Autodesk Fusion 360 part; units mm, degrees
(part 2 of 3)
sketch "Sketch3" plane through (0, 0, 0) normal (0, -1, 0) x (1, 0, 0)
  spline S0 degree 3 poles (-0.0363, -10.6479) (-0.1747, -12.1181) (-0.1574, -12.2391) (0.1193, -12.2391) knots -1 -1 -1 -1 0 0 0 0
  spline S1 degree 3 poles (0.0329, -8.3995) (0.0674, -8.7454) (0.0329, -9.7659) (-0.0363, -10.6479) knots -1 -1 -1 -1 0 0 0 0
  spline S2 degree 3 poles (0.6036, -7.6558) (-0.0363, -7.7596) (-0.0536, -7.7769) (0.0329, -8.3995) knots -1 -1 -1 -1 0 0 0 0
  spline S3 degree 3 poles (1.9872, -8.5379) (1.9872, -7.8288) (1.4857, -7.5002) (0.6036, -7.6558) knots -1 -1 -1 -1 0 0 0 0
  spline S4 degree 3 poles (2.091, -10.6479) (2.0391, -9.7832) (1.9872, -8.8319) (1.9872, -8.5379) knots -1 -1 -1 -1 0 0 0 0
  spline S5 degree 3 poles (1.8316, -12.2391) (2.1948, -12.2391) (2.2121, -12.1872) (2.091, -10.6479) knots -1 -1 -1 -1 0 0 0 0
  spline S6 degree 3 poles (1.4684, -11.5646) (1.4684, -12.1353) (1.5203, -12.2391) (1.8316, -12.2391) knots -1 -1 -1 -1 0 0 0 0
  spline S7 degree 3 poles (0.6901, -10.6825) (1.0879, -10.3539) (1.4684, -10.769) (1.4684, -11.5646) knots -1 -1 -1 -1 0 0 0 0
  spline S8 degree 3 poles (0.4306, -11.5646) (0.4306, -11.1841) (0.5344, -10.8036) (0.6901, -10.6825) knots -1 -1 -1 -1 0 0 0 0
  spline S9 degree 3 poles (0.1193, -12.2391) (0.3615, -12.2391) (0.4306, -12.1008) (0.4306, -11.5646) knots -1 -1 -1 -1 0 0 0 0
  spline S10 degree 3 poles (4.9966, -12.0835) (5.1869, -12.2737) (10.1161, -11.7548) (10.1161, -11.5473) knots -1 -1 -1 -1 0 0 0 0
  spline S11 degree 3 poles (4.9275, -11.4435) (4.9275, -11.7548) (4.962, -12.0489) (4.9966, -12.0835) knots -1 -1 -1 -1 0 0 0 0
  spline S12 degree 3 poles (5.4117, -10.942) (4.962, -10.8728) (4.9275, -10.9074) (4.9275, -11.4435) knots -1 -1 -1 -1 0 0 0 0
  spline S13 degree 3 poles (7.3488, -11.1149) (6.5359, -11.063) (5.6712, -10.9766) (5.4117, -10.942) knots -1 -1 -1 -1 0 0 0 0
  spline S14 degree 3 poles (10.1161, -11.5473) (10.1161, -11.3916) (9.2167, -11.236) (7.3488, -11.1149) knots -1 -1 -1 -1 0 0 0 0
  spline S15 degree 3 poles (-0.3304, -6.5316) (0.1885, -6.6873) (1.1916, -6.6008) (1.624, -6.3587) knots -1 -1 -1 -1 0 0 0 0
  spline S16 degree 3 poles (-1.9215, -5.0269) (-1.6275, -5.7187) (-0.9876, -6.3241) (-0.3304, -6.5316) knots -1 -1 -1 -1 0 0 0 0
  spline S17 degree 3 poles (-1.5929, -3.8681) (-2.2329, -4.1449) (-2.2674, -4.2313) (-1.9215, -5.0269) knots -1 -1 -1 -1 0 0 0 0
  spline S18 degree 3 poles (-0.4514, -2.4499) (-0.192, -2.7612) (-0.8146, -3.5568) (-1.5929, -3.8681) knots -1 -1 -1 -1 0 0 0 0
  spline S19 degree 3 poles (-1.5064, -2.6402) (-0.9184, -2.1386) (-0.7281, -2.104) (-0.4514, -2.4499) knots -1 -1 -1 -1 0 0 0 0
  spline S20 degree 3 poles (-3.7376, -2.571) (-3.0803, -3.2282) (-2.2328, -3.2455) (-1.5064, -2.6402) knots -1 -1 -1 -1 0 0 0 0
  spline S21 degree 3 poles (-4.2391, -1.81) (-4.2391, -1.9483) (-4.0143, -2.2943) (-3.7376, -2.571) knots -1 -1 -1 -1 0 0 0 0
  spline S22 degree 3 poles (-5.0693, -1.5851) (-4.7753, -1.2911) (-4.2391, -1.4295) (-4.2391, -1.81) knots -1 -1 -1 -1 0 0 0 0
  spline S23 degree 3 poles (-3.8932, -3.7471) (-4.7753, -3.2455) (-5.4671, -1.9829) (-5.0693, -1.5851) knots -1 -1 -1 -1 0 0 0 0
  spline S24 degree 3 poles (-4.8445, -5.4939) (-3.2187, -5.4939) (-2.6479, -4.4389) (-3.8932, -3.7471) knots -1 -1 -1 -1 0 0 0 0
  spline S25 degree 3 poles (-6.574, -4.387) (-7.1966, -4.6291) (-5.8476, -5.4939) (-4.8445, -5.4939) knots -1 -1 -1 -1 0 0 0 0
  spline S26 degree 3 poles (-6.3492, -3.9027) (-6.3146, -4.1276) (-6.401, -4.3351) (-6.574, -4.387) knots -1 -1 -1 -1 0 0 0 0
  spline S27 degree 3 poles (-7.0929, -3.5568) (-6.4875, -3.5049) (-6.401, -3.5568) (-6.3492, -3.9027) knots -1 -1 -1 -1 0 0 0 0
  spline S28 degree 3 poles (-10.2233, -1.7581) (-9.7045, -3.1071) (-8.7186, -3.6606) (-7.0929, -3.5568) knots -1 -1 -1 -1 0 0 0 0
  spline S29 degree 3 poles (-10.3098, -0.3053) (-10.4828, -0.876) (-10.4655, -1.1009) (-10.2233, -1.7581) knots -1 -1 -1 -1 0 0 0 0
  spline S30 degree 3 poles (-8.2171, 1.701) (-9.0645, 1.5626) (-10.0158, 0.6633) (-10.3098, -0.3053) knots -1 -1 -1 -1 0 0 0 0
  spline S31 degree 3 poles (-7.3523, 2.5312) (-7.041, 2.168) (-7.3869, 1.8394) (-8.2171, 1.701) knots -1 -1 -1 -1 0 0 0 0
  spline S32 degree 3 poles (-7.923, 2.8425) (-7.7155, 2.8079) (-7.4561, 2.6695) (-7.3523, 2.5312) knots -1 -1 -1 -1 0 0 0 0
  spline S33 degree 3 poles (-7.8366, 3.3613) (-8.3035, 2.8944) (-8.3035, 2.8944) (-7.923, 2.8425) knots -1 -1 -1 -1 0 0 0 0
  spline S34 degree 3 poles (-6.6778, 3.8456) (-7.1966, 3.8456) (-7.4734, 3.7246) (-7.8366, 3.3613) knots -1 -1 -1 -1 0 0 0 0
  line L0 (-6.6778, 3.8456) -> (-5.9687, 3.8456)
  line L1 (-5.9687, 3.8456) -> (-6.3319, 3.1711)
  spline S35 degree 3 poles (-6.1416, 1.5107) (-6.7297, 1.5107) (-6.7988, 2.2544) (-6.3319, 3.1711) knots -1 -1 -1 -1 0 0 0 0
  spline S36 degree 3 poles (-5.6055, 2.1161) (-5.7092, 1.6145) (-5.7957, 1.5107) (-6.1416, 1.5107) knots -1 -1 -1 -1 0 0 0 0
  spline S37 degree 3 poles (-5.0001, 3.1192) (-5.2595, 2.8944) (-5.5363, 2.4447) (-5.6055, 2.1161) knots -1 -1 -1 -1 0 0 0 0
  spline S38 degree 3 poles (-3.5646, 3.4651) (-4.3775, 3.517) (-4.6196, 3.4651) (-5.0001, 3.1192) knots -1 -1 -1 -1 0 0 0 0
  spline S39 degree 3 poles (-2.5442, 3.7764) (-2.5961, 3.4478) (-2.6825, 3.4132) (-3.5646, 3.4651) knots -1 -1 -1 -1 0 0 0 0
  spline S40 degree 3 poles (-4.3083, 4.5028) (-3.3052, 4.6066) (-2.475, 4.278) (-2.5442, 3.7764) knots -1 -1 -1 -1 0 0 0 0
  spline S41 degree 3 poles (-4.4121, 5.6962) (-5.813, 4.9525) (-5.7611, 4.3299) (-4.3083, 4.5028) knots -1 -1 -1 -1 0 0 0 0
  spline S42 degree 3 poles (-1.5929, 5.8519) (-2.4404, 6.2151) (-3.5646, 6.1459) (-4.4121, 5.6962) knots -1 -1 -1 -1 0 0 0 0
  spline S43 degree 3 poles (0.0847, 4.1223) (0.0847, 4.5028) (-0.9876, 5.6098) (-1.5929, 5.8519) knots -1 -1 -1 -1 0 0 0 0
  spline S44 degree 3 poles (0.8457, 3.6035) (0.5171, 3.4824) (0.0847, 3.7764) (0.0847, 4.1223) knots -1 -1 -1 -1 0 0 0 0
  spline S45 degree 3 poles (0.8457, 4.9179) (1.1916, 4.2261) (1.1916, 3.7418) (0.8457, 3.6035) knots -1 -1 -1 -1 0 0 0 0
  spline S46 degree 3 poles (0.863, 5.6789) (0.5863, 5.4714) (0.5863, 5.4195) (0.8457, 4.9179) knots -1 -1 -1 -1 0 0 0 0
  spline S47 degree 3 poles (3.4055, 6.0075) (2.7136, 6.1459) (1.2608, 5.973) (0.863, 5.6789) knots -1 -1 -1 -1 0 0 0 0
  spline S48 degree 3 poles (4.6334, 5.5406) (4.2702, 5.7308) (3.7168, 5.9384) (3.4055, 6.0075) knots -1 -1 -1 -1 0 0 0 0
  spline S49 degree 3 poles (4.9966, 4.866) (5.2907, 5.1947) (5.2907, 5.212) (4.6334, 5.5406) knots -1 -1 -1 -1 0 0 0 0
  spline S50 degree 3 poles (4.2875, 4.5374) (4.5124, 4.5374) (4.841, 4.6931) (4.9966, 4.866) knots -1 -1 -1 -1 0 0 0 0
  spline S51 degree 3 poles (2.5407, 3.811) (2.8347, 4.1396) (3.7687, 4.5374) (4.2875, 4.5374) knots -1 -1 -1 -1 0 0 0 0
  spline S52 degree 3 poles (2.8347, 2.9808) (2.4369, 2.9808) (2.2813, 3.4824) (2.5407, 3.811) knots -1 -1 -1 -1 0 0 0 0
  spline S53 degree 3 poles (3.44, 3.2403) (3.2671, 3.1019) (2.9904, 2.9808) (2.8347, 2.9808) knots -1 -1 -1 -1 0 0 0 0
  spline S54 degree 3 poles (6.2073, 2.2026) (5.9479, 3.2576) (4.2875, 3.8802) (3.44, 3.2403) knots -1 -1 -1 -1 0 0 0 0
  spline S55 degree 3 poles (6.6743, 1.7702) (6.4322, 1.7702) (6.2765, 1.9258) (6.2073, 2.2026) knots -1 -1 -1 -1 0 0 0 0
  spline S56 degree 3 poles (6.3803, 3.7937) (7.2796, 2.929) (7.4526, 1.7702) (6.6743, 1.7702) knots -1 -1 -1 -1 0 0 0 0
  line L2 (6.3803, 3.7937) -> (5.7749, 4.3472)
  line L3 (5.7749, 4.3472) -> (6.3284, 4.6412)
  spline S57 degree 3 poles (9.2686, 4.2607) (8.5941, 4.9006) (7.1931, 5.0736) (6.3284, 4.6412) knots -1 -1 -1 -1 0 0 0 0
  spline S58 degree 3 poles (9.4243, 3.6381) (9.7702, 3.7591) (9.7702, 3.7937) (9.2686, 4.2607) knots -1 -1 -1 -1 0 0 0 0
  spline S59 degree 3 poles (9.1129, 3.1192) (9.0783, 3.3786) (9.1648, 3.5516) (9.4243, 3.6381) knots -1 -1 -1 -1 0 0 0 0
  spline S60 degree 3 poles (9.9604, 2.7733) (9.2513, 2.7214) (9.1648, 2.756) (9.1129, 3.1192) knots -1 -1 -1 -1 0 0 0 0
  spline S61 degree 3 poles (11.7764, 0.473) (12.2953, 1.7183) (11.3959, 2.8598) (9.9604, 2.7733) knots -1 -1 -1 -1 0 0 0 0
  spline S62 degree 3 poles (11.2403, -0.2361) (11.3959, -0.1842) (11.6381, 0.1444) (11.7764, 0.473) knots -1 -1 -1 -1 0 0 0 0
  spline S63 degree 3 poles (10.9808, -0.755) (10.9808, -0.5301) (11.1019, -0.288) (11.2403, -0.2361) knots -1 -1 -1 -1 0 0 0 0
  spline S64 degree 3 poles (12.278, -0.6512) (11.6554, -1.3084) (10.9808, -1.3603) (10.9808, -0.755) knots -1 -1 -1 -1 0 0 0 0
  spline S65 degree 3 poles (13.0563, -1.2219) (13.0563, -0.1842) (12.8487, -0.0459) (12.278, -0.6512) knots -1 -1 -1 -1 0 0 0 0
  spline S66 degree 3 poles (12.2261, -3.1071) (12.8487, -2.4326) (13.0563, -1.9829) (13.0563, -1.2219) knots -1 -1 -1 -1 0 0 0 0
  spline S67 degree 3 poles (9.0092, -2.8823) (9.8566, -3.8854) (11.3959, -4.0065) (12.2261, -3.1071) knots -1 -1 -1 -1 0 0 0 0
  spline S68 degree 3 poles (8.1098, -3.4185) (7.5218, -2.4326) (8.2655, -2.0002) (9.0092, -2.8823) knots -1 -1 -1 -1 0 0 0 0
  spline S69 degree 3 poles (8.3865, -4.093) (8.3865, -3.9892) (8.2655, -3.6952) (8.1098, -3.4185) knots -1 -1 -1 -1 0 0 0 0
  spline S70 degree 3 poles (6.7089, -5.7706) (7.2796, -5.5458) (8.3865, -4.4216) (8.3865, -4.093) knots -1 -1 -1 -1 0 0 0 0
  spline S71 degree 3 poles (4.4086, -5.8398) (4.8583, -6.082) (6.0516, -6.0474) (6.7089, -5.7706) knots -1 -1 -1 -1 0 0 0 0
  spline S72 degree 3 poles (4.5124, -5.0269) (4.0973, -5.6323) (4.0973, -5.6669) (4.4086, -5.8398) knots -1 -1 -1 -1 0 0 0 0
  spline S73 degree 3 poles (4.4951, -3.332) (5.0312, -3.332) (5.0485, -4.2313) (4.5124, -5.0269) knots -1 -1 -1 -1 0 0 0 0
  spline S74 degree 3 poles (3.9589, -3.92) (4.0973, -3.5049) (4.2529, -3.332) (4.4951, -3.332) knots -1 -1 -1 -1 0 0 0 0
  spline S75 degree 3 poles (1.2781, -4.7675) (2.2985, -5.5285) (3.5784, -5.1307) (3.9589, -3.92) knots -1 -1 -1 -1 0 0 0 0
  spline S76 degree 3 poles (0.4998, -4.6637) (0.742, -4.4043) (0.8111, -4.4216) (1.2781, -4.7675) knots -1 -1 -1 -1 0 0 0 0
  spline S77 degree 3 poles (1.2262, -5.9263) (0.4133, -5.5285) (0.1193, -5.0442) (0.4998, -4.6637) knots -1 -1 -1 -1 0 0 0 0
  spline S78 degree 3 poles (1.624, -6.3587) (1.797, -6.2722) (1.6932, -6.1511) (1.2262, -5.9263) knots -1 -1 -1 -1 0 0 0 0
  spline S79 degree 3 poles (3.1287, -11.703) (3.2152, -12.0835) (3.3363, -12.2391) (3.5957, -12.2391) knots -1 -1 -1 -1 0 0 0 0
  spline S80 degree 3 poles (3.025, -9.714) (3.025, -10.5096) (3.0768, -11.4089) (3.1287, -11.703) knots -1 -1 -1 -1 0 0 0 0
  spline S81 degree 3 poles (3.3709, -8.2612) (3.0595, -8.2612) (3.025, -8.3822) (3.025, -9.714) knots -1 -1 -1 -1 0 0 0 0
  spline S82 degree 3 poles (3.7168, -9.0914) (3.7168, -8.3822) (3.6649, -8.2612) (3.3709, -8.2612) knots -1 -1 -1 -1 0 0 0 0
  spline S83 degree 3 poles (3.8378, -11.0803) (3.7687, -10.4231) (3.7168, -9.541) (3.7168, -9.0914) knots -1 -1 -1 -1 0 0 0 0
  spline S84 degree 3 poles (3.5957, -12.2391) (3.9243, -12.2391) (3.9243, -12.1699) (3.8378, -11.0803) knots -1 -1 -1 -1 0 0 0 0
  spline S85 degree 3 poles (-8.1133, -5.6669) (-7.8366, -5.8571) (-7.4388, -6.0128) (-7.2312, -6.0128) knots -1 -1 -1 -1 0 0 0 0
  spline S86 degree 3 poles (-8.8743, -4.8713) (-8.7359, -5.1307) (-8.4073, -5.4939) (-8.1133, -5.6669) knots -1 -1 -1 -1 0 0 0 0
  line L4 (-8.8743, -4.8713) -> (-9.1164, -4.4043)
  line L5 (-9.1164, -4.4043) -> (-8.5457, -4.5254)
  spline S87 degree 3 poles (-7.8885, -4.854) (-7.923, -4.7329) (-8.2171, -4.5772) (-8.5457, -4.5254) knots -1 -1 -1 -1 0 0 0 0
  spline S88 degree 3 poles (-7.335, -5.5285) (-7.5944, -5.2691) (-7.8539, -4.9577) (-7.8885, -4.854) knots -1 -1 -1 -1 0 0 0 0
  spline S89 degree 3 poles (-7.2312, -6.0128) (-6.868, -6.0128) (-6.8853, -5.9955) (-7.335, -5.5285) knots -1 -1 -1 -1 0 0 0 0
  spline S90 degree 3 poles (2.5061, -7.1024) (2.5061, -7.3272) (3.4919, -7.2234) (3.6995, -6.9986) knots -1 -1 -1 -1 0 0 0 0
  spline S91 degree 3 poles (2.7828, -6.6873) (2.6272, -6.8602) (2.5061, -7.0505) (2.5061, -7.1024) knots -1 -1 -1 -1 0 0 0 0
  spline S92 degree 3 poles (3.4746, -6.5662) (3.1287, -6.4106) (3.0077, -6.4452) (2.7828, -6.6873) knots -1 -1 -1 -1 0 0 0 0
  spline S93 degree 3 poles (3.6995, -6.9986) (3.8378, -6.8084) (3.786, -6.7219) (3.4746, -6.5662) knots -1 -1 -1 -1 0 0 0 0
  spline S94 degree 3 poles (10.8771, 3.7937) (11.3613, 3.2576) (11.4997, 3.223) (11.4997, 3.5862) knots -1 -1 -1 -1 0 0 0 0
  spline S95 degree 3 poles (10.5485, 4.3299) (10.4966, 4.278) (10.6522, 4.0359) (10.8771, 3.7937) knots -1 -1 -1 -1 0 0 0 0
  spline S96 degree 3 poles (11.4997, 3.5862) (11.4997, 3.8456) (10.6868, 4.4683) (10.5485, 4.3299) knots -1 -1 -1 -1 0 0 0 0
  line L6 (-7.4388, 4.9006) -> (-7.0237, 5.2293)
  spline S97 degree 3 poles (-6.4875, 5.2293) (-6.2454, 5.6789) (-6.5048, 5.6789) (-7.0237, 5.2293) knots -1 -1 -1 -1 0 0 0 0
  spline S98 degree 3 poles (-7.0583, 4.8833) (-6.8507, 4.8833) (-6.5913, 5.039) (-6.4875, 5.2293) knots -1 -1 -1 -1 0 0 0 0
  line L7 (-7.0583, 4.8833) -> (-7.4388, 4.9006)
  spline S99 degree 3 poles (-1.0222, 6.6129) (-0.7454, 6.4399) (-0.4341, 6.2843) (-0.3477, 6.2843) knots -1 -1 -1 -1 0 0 0 0
  line L8 (-1.0222, 6.6129) -> (-1.5064, 6.9242)
  line L9 (-1.5064, 6.9242) -> (-1.0741, 7.2009)
  spline S100 degree 3 poles (1.2089, 7.4085) (0.4479, 7.7198) (-0.4168, 7.6506) (-1.0741, 7.2009) knots -1 -1 -1 -1 0 0 0 0
  spline S101 degree 3 poles (1.7624, 7.0107) (1.8143, 7.0799) (1.5721, 7.2528) (1.2089, 7.4085) knots -1 -1 -1 -1 0 0 0 0
  spline S102 degree 3 poles (-0.3477, 6.2843) (-0.1228, 6.2843) (1.624, 6.8723) (1.7624, 7.0107) knots -1 -1 -1 -1 0 0 0 0
  spline S103 degree 3 poles (-3.7203, -12.0662) (-1.2816, -12.2737) (-1.2297, -12.2564) (-1.1605, -11.4954) knots -1 -1 -1 -1 0 0 0 0
  spline S104 degree 3 poles (-7.0064, -11.53) (-7.0064, -11.703) (-5.9341, -11.8759) (-3.7203, -12.0662) knots -1 -1 -1 -1 0 0 0 0
  spline S105 degree 3 poles (-6.8507, -11.3743) (-6.9372, -11.3743) (-7.0064, -11.4435) (-7.0064, -11.53) knots -1 -1 -1 -1 0 0 0 0
  spline S106 degree 3 poles (-5.4152, -11.2187) (-6.107, -11.3052) (-6.7642, -11.3743) (-6.8507, -11.3743) knots -1 -1 -1 -1 0 0 0 0
  spline S107 degree 3 poles (-2.6306, -10.942) (-3.4608, -11.0111) (-4.7234, -11.1322) (-5.4152, -11.2187) knots -1 -1 -1 -1 0 0 0 0
  line L10 (-2.6306, -10.942) -> (-1.1086, -10.8382)
  line L11 (-1.1086, -10.8382) -> (-1.1605, -11.4954)
  spline S108 degree 3 poles (-3.5473, -7.258) (-3.2187, -7.431) (-2.8728, -7.5694) (-2.8036, -7.5694) knots -1 -1 -1 -1 0 0 0 0
  spline S109 degree 3 poles (-3.4435, -6.203) (-4.3083, -6.5835) (-4.3429, -6.8775) (-3.5473, -7.258) knots -1 -1 -1 -1 0 0 0 0
  line L12 (-3.4435, -6.203) -> (-2.7344, -5.8744)
  line L13 (-2.7344, -5.8744) -> (-2.2674, -6.4797)
  spline S110 degree 3 poles (-1.8524, -7.1197) (-1.8178, -7.1024) (-1.9907, -6.8084) (-2.2674, -6.4797) knots -1 -1 -1 -1 0 0 0 0
  spline S111 degree 3 poles (-2.8036, -7.5694) (-2.6825, -7.5694) (-1.9907, -7.258) (-1.8524, -7.1197) knots -1 -1 -1 -1 0 0 0 0
  spline S112 degree 3 poles (8.6979, -6.2203) (9.4588, -6.3933) (10.6349, -5.6842) (10.6349, -5.0615) knots -1 -1 -1 -1 0 0 0 0
  spline S113 degree 3 poles (8.8535, -5.3555) (8.3001, -6.0992) (8.3001, -6.1338) (8.6979, -6.2203) knots -1 -1 -1 -1 0 0 0 0
  spline S114 degree 3 poles (9.3551, -4.6637) (9.3378, -4.6983) (9.1129, -5.0096) (8.8535, -5.3555) knots -1 -1 -1 -1 0 0 0 0
  spline S115 degree 3 poles (10.6349, -5.0615) (10.6349, -4.8713) (9.4589, -4.5081) (9.3551, -4.6637) knots -1 -1 -1 -1 0 0 0 0
  spline S116 degree 3 poles (-2.769, -20.956) (-1.0395, -21.0598) (6.8127, -20.9041) (8.5595, -20.7139) knots -1 -1 -1 -1 0 0 0 0
  spline S117 degree 3 poles (-9.6526, -20.0221) (-9.9293, -20.2642) (-6.6432, -20.7139) (-2.769, -20.956) knots -1 -1 -1 -1 0 0 0 0
  spline S118 degree 3 poles (-5.8822, -19.4167) (-7.5771, -19.5378) (-9.4623, -19.8491) (-9.6526, -20.0221) knots -1 -1 -1 -1 0 0 0 0
  spline S119 degree 3 poles (-4.1181, -19.2265) (-4.3256, -19.2784) (-5.1212, -19.3475) (-5.8822, -19.4167) knots -1 -1 -1 -1 0 0 0 0
  spline S120 degree 3 poles (-3.6338, -19.5205) (-3.703, -19.2611) (-3.8586, -19.1746) (-4.1181, -19.2265) knots -1 -1 -1 -1 0 0 0 0
  spline S121 degree 3 poles (-3.1495, -19.8145) (-3.3916, -19.8491) (-3.5473, -19.7626) (-3.6338, -19.5205) knots -1 -1 -1 -1 0 0 0 0
  spline S122 degree 3 poles (-0.7281, -14.8507) (-1.2124, -16.8743) (-2.6133, -19.7453) (-3.1495, -19.8145) knots -1 -1 -1 -1 0 0 0 0
  spline S123 degree 3 poles (0.0501, -13.2768) (-0.3131, -13.2768) (-0.3822, -13.4325) (-0.7281, -14.8507) knots -1 -1 -1 -1 0 0 0 0
  spline S124 degree 3 poles (0.3615, -14.1935) (0.4479, -13.3287) (0.4306, -13.2768) (0.0501, -13.2768) knots -1 -1 -1 -1 0 0 0 0
  spline S125 degree 3 poles (-0.019, -19.5897) (-0.1055, -19.3648) (0.0329, -17.2894) (0.3615, -14.1935) knots -1 -1 -1 -1 0 0 0 0
  spline S126 degree 3 poles (0.742, -19.5551) (0.5517, -19.9183) (0.102, -19.9356) (-0.019, -19.5897) knots -1 -1 -1 -1 0 0 0 0
  spline S127 degree 3 poles (1.1052, -17.1683) (1.0014, -18.3098) (0.8284, -19.3821) (0.742, -19.5551) knots -1 -1 -1 -1 0 0 0 0
  spline S128 degree 3 poles (1.8316, -13.2768) (1.4684, -13.2768) (1.4684, -13.1904) (1.1052, -17.1683) knots -1 -1 -1 -1 0 0 0 0
  spline S129 degree 3 poles (2.1602, -13.4152) (2.1602, -13.3287) (2.0045, -13.2768) (1.8316, -13.2768) knots -1 -1 -1 -1 0 0 0 0
  spline S130 degree 3 poles (2.679, -17.8774) (2.558, -17.5661) (2.1602, -14.1416) (2.1602, -13.4152) knots -1 -1 -1 -1 0 0 0 0
  spline S131 degree 3 poles (3.5957, -18.0677) (3.44, -18.4482) (2.852, -18.3271) (2.679, -17.8774) knots -1 -1 -1 -1 0 0 0 0
  spline S132 degree 3 poles (3.5438, -17.0645) (3.613, -17.4969) (3.6476, -17.9293) (3.5957, -18.0677) knots -1 -1 -1 -1 0 0 0 0
  spline S133 degree 3 poles (3.2844, -14.7988) (3.3536, -15.629) (3.4746, -16.6494) (3.5438, -17.0645) knots -1 -1 -1 -1 0 0 0 0
  line L14 (3.2844, -14.7988) -> (3.1633, -13.2768)
  line L15 (3.1633, -13.2768) -> (3.6995, -13.2768)
  spline S134 degree 3 poles (4.2356, -13.6746) (4.2356, -13.346) (4.1492, -13.2768) (3.6995, -13.2768) knots -1 -1 -1 -1 0 0 0 0
  spline S135 degree 3 poles (5.3771, -17.7736) (4.8929, -16.684) (4.2356, -14.3492) (4.2356, -13.6746) knots -1 -1 -1 -1 0 0 0 0
  spline S136 degree 3 poles (6.3284, -19.2611) (6.0517, -18.9843) (5.6193, -18.3271) (5.3771, -17.7736) knots -1 -1 -1 -1 0 0 0 0
  spline S137 degree 3 poles (7.0894, -19.5032) (6.8645, -19.6934) (6.7435, -19.6588) (6.3284, -19.2611) knots -1 -1 -1 -1 0 0 0 0
  spline S138 degree 3 poles (8.7324, -19.3821) (7.7293, -19.3129) (7.2796, -19.3475) (7.0894, -19.5032) knots -1 -1 -1 -1 0 0 0 0
  spline S139 degree 3 poles (12.3645, -20.0221) (12.3645, -19.8491) (10.5139, -19.5205) (8.7324, -19.3821) knots -1 -1 -1 -1 0 0 0 0
  spline S140 degree 3 poles (8.5595, -20.7139) (10.6868, -20.5063) (12.3645, -20.195) (12.3645, -20.0221) knots -1 -1 -1 -1 0 0 0 0
  spline S141 degree 3 poles (-11.2957, -19.901) (-11.5032, -20.9733) (-9.3067, -21.5613) (-3.7894, -21.9246) knots 0 0 0 0 1 1 1 1
  spline S142 degree 3 poles (-3.7894, -21.9246) (-1.0568, -22.0975) (6.6743, -21.9937) (8.9054, -21.7343) knots 0 0 0 0 1 1 1 1
  spline S143 degree 3 poles (8.9054, -21.7343) (10.9117, -21.5095) (12.7277, -21.1463) (13.3676, -20.8522) knots 0 0 0 0 1 1 1 1
  spline S144 degree 3 poles (13.3676, -20.8522) (13.9384, -20.5755) (14.0767, -19.8664) (13.627, -19.4513) knots 0 0 0 0 1 1 1 1
  spline S145 degree 3 poles (13.627, -19.4513) (13.0736, -18.967) (10.7906, -18.5346) (7.2623, -18.2406) knots 0 0 0 0 1 1 1 1
  spline S146 degree 3 poles (7.2623, -18.2406) (6.8645, -18.2233) (6.6743, -18.0504) (6.363, -17.5142) knots 0 0 0 0 1 1 1 1
  spline S147 degree 3 poles (6.363, -17.5142) (5.9825, -16.8224) (5.3425, -14.6605) (5.2388, -13.7092) knots 0 0 0 0 1 1 1 1
  spline S148 degree 3 poles (5.2388, -13.7092) (5.1869, -13.2077) (5.2215, -13.1904) (5.8787, -13.1558) knots 0 0 0 0 1 1 1 1
  spline S149 degree 3 poles (5.8787, -13.1558) (7.4872, -13.052) (9.9258, -12.7234) (10.756, -12.4813) knots 0 0 0 0 1 1 1 1
  spline S150 degree 3 poles (10.756, -12.4813) (12.1223, -12.1008) (12.3645, -11.3052) (11.3095, -10.7517) knots 0 0 0 0 1 1 1 1
  spline S151 degree 3 poles (11.3095, -10.7517) (10.756, -10.475) (8.2136, -10.0599) (6.1035, -9.8869) knots 0 0 0 0 1 1 1 1
  line L16 (6.1035, -9.8869) -> (4.7891, -9.7832)
  line L17 (4.7891, -9.7832) -> (4.7199, -8.7281)
  spline S152 degree 3 poles (4.7199, -8.7281) (4.6507, -7.431) (4.8237, -7.0505) (5.5501, -7.0505) knots 0 0 0 0 1 1 1 1
  spline S153 degree 3 poles (5.5501, -7.0505) (5.8441, -7.0505) (6.3284, -6.964) (6.6397, -6.8602) knots 0 0 0 0 1 1 1 1
  spline S154 degree 3 poles (6.6397, -6.8602) (7.0721, -6.7046) (7.2969, -6.7219) (7.7639, -6.9467) knots 0 0 0 0 1 1 1 1
  spline S155 degree 3 poles (7.7639, -6.9467) (8.5768, -7.3272) (9.7356, -7.2926) (10.4274, -6.8775) knots 0 0 0 0 1 1 1 1
  spline S156 degree 3 poles (10.4274, -6.8775) (11.05, -6.497) (11.6727, -5.5977) (11.6727, -5.0615) knots 0 0 0 0 1 1 1 1
  spline S157 degree 3 poles (11.6727, -5.0615) (11.6727, -4.8367) (11.9321, -4.5772) (12.3645, -4.3178) knots 0 0 0 0 1 1 1 1
  spline S158 degree 3 poles (12.3645, -4.3178) (14.0248, -3.3839) (14.4918, -1.3949) (13.4887, 0.3001) knots 0 0 0 0 1 1 1 1
  spline S159 degree 3 poles (13.4887, 0.3001) (12.8833, 1.3032) (12.6758, 1.9777) (12.6931, 2.7906) knots 0 0 0 0 1 1 1 1
  spline S160 degree 3 poles (12.6931, 2.7906) (12.7277, 3.6035) (12.1396, 4.745) (11.4997, 5.1082) knots 0 0 0 0 1 1 1 1
  spline S161 degree 3 poles (11.4997, 5.1082) (11.1538, 5.3157) (10.6868, 5.4195) (10.1507, 5.3849) knots 0 0 0 0 1 1 1 1
  spline S162 degree 3 poles (10.1507, 5.3849) (9.701, 5.3676) (9.1129, 5.4541) (8.8189, 5.5579) knots 0 0 0 0 1 1 1 1
  spline S163 degree 3 poles (8.8189, 5.5579) (8.5422, 5.6789) (7.8158, 5.7481) (7.245, 5.7135) knots 0 0 0 0 1 1 1 1
  spline S164 degree 3 poles (7.245, 5.7135) (6.6397, 5.6962) (6.0862, 5.7481) (5.9479, 5.8519) knots 0 0 0 0 1 1 1 1
  spline S165 degree 3 poles (5.9479, 5.8519) (5.4982, 6.2151) (4.2529, 6.7858) (3.907, 6.7858) knots 0 0 0 0 1 1 1 1
  spline S166 degree 3 poles (3.907, 6.7858) (3.7168, 6.7858) (3.2844, 7.0453) (2.9731, 7.3739) knots 0 0 0 0 1 1 1 1
  spline S167 degree 3 poles (2.9731, 7.3739) (1.624, 8.7229) (-0.0363, 8.9824) (-1.5237, 8.1176) knots 0 0 0 0 1 1 1 1
  spline S168 degree 3 poles (-1.5237, 8.1176) (-1.9907, 7.8409) (-2.4058, 7.5122) (-2.4577, 7.3739) knots 0 0 0 0 1 1 1 1
  spline S169 degree 3 poles (-2.4577, 7.3739) (-2.5096, 7.2355) (-2.7863, 7.1317) (-3.0976, 7.1317) knots 0 0 0 0 1 1 1 1
  spline S170 degree 3 poles (-3.0976, 7.1317) (-3.3916, 7.1145) (-3.9451, 6.9934) (-4.3256, 6.8377) knots 0 0 0 0 1 1 1 1
  spline S171 degree 3 poles (-4.3256, 6.8377) (-4.7061, 6.6994) (-5.3806, 6.5956) (-5.8303, 6.5956) knots 0 0 0 0 1 1 1 1
  spline S172 degree 3 poles (-5.8303, 6.5956) (-6.2973, 6.6129) (-6.9199, 6.5091) (-7.2831, 6.3362) knots 0 0 0 0 1 1 1 1
  spline S173 degree 3 poles (-7.2831, 6.3362) (-7.9749, 6.0075) (-8.7359, 5.0044) (-8.7359, 4.4164) knots 0 0 0 0 1 1 1 1
  spline S174 degree 3 poles (-8.7359, 4.4164) (-8.7359, 4.2088) (-8.8916, 3.7764) (-9.0818, 3.4651) knots 0 0 0 0 1 1 1 1
  spline S175 degree 3 poles (-9.0818, 3.4651) (-9.2721, 3.1538) (-9.4277, 2.7733) (-9.4277, 2.6349) knots 0 0 0 0 1 1 1 1
  spline S176 degree 3 poles (-9.4277, 2.6349) (-9.445, 2.4966) (-9.7391, 2.168) (-10.1023, 1.9258) knots 0 0 0 0 1 1 1 1
  spline S177 degree 3 poles (-10.1023, 1.9258) (-10.9497, 1.3205) (-11.3994, 0.3865) (-11.3994, -0.8241) knots 0 0 0 0 1 1 1 1
  spline S178 degree 3 poles (-11.3994, -0.8241) (-11.3821, -1.7927) (-10.9324, -2.9515) (-10.3963, -3.4012) knots 0 0 0 0 1 1 1 1
  spline S179 degree 3 poles (-10.3963, -3.4012) (-10.2406, -3.5395) (-10.1196, -3.8335) (-10.1196, -4.093) knots 0 0 0 0 1 1 1 1
  spline S180 degree 3 poles (-10.1196, -4.093) (-10.1023, -4.9059) (-9.4969, -5.9609) (-8.7186, -6.4797) knots 0 0 0 0 1 1 1 1
  spline S181 degree 3 poles (-8.7186, -6.4797) (-8.1306, -6.8775) (-7.802, -6.964) (-7.0237, -6.9467) knots 0 0 0 0 1 1 1 1
  spline S182 degree 3 poles (-7.0237, -6.9467) (-6.4875, -6.9467) (-5.8995, -6.8948) (-5.7092, -6.8257) knots 0 0 0 0 1 1 1 1
  spline S183 degree 3 poles (-5.7092, -6.8257) (-5.4325, -6.7219) (-5.2768, -6.8257) (-4.9828, -7.2926) knots 0 0 0 0 1 1 1 1
  spline S184 degree 3 poles (-4.9828, -7.2926) (-4.2564, -8.4168) (-2.7171, -8.8146) (-1.5064, -8.192) knots 0 0 0 0 1 1 1 1
  line L18 (-1.5064, -8.192) -> (-0.953, -7.898)
  line L19 (-0.953, -7.898) -> (-0.953, -9.7832)
  line L20 (-0.953, -9.7832) -> (-2.4577, -9.8869)
  spline S185 degree 3 poles (-2.4577, -9.8869) (-4.9309, -10.0599) (-7.6463, -10.475) (-8.1825, -10.7517) knots 0 0 0 0 1 1 1 1
  spline S186 degree 3 poles (-8.1825, -10.7517) (-9.0991, -11.236) (-9.0818, -11.8586) (-8.1133, -12.3256) knots 0 0 0 0 1 1 1 1
  spline S187 degree 3 poles (-8.1133, -12.3256) (-7.4388, -12.6369) (-4.3083, -13.1039) (-2.7171, -13.1039) knots 0 0 0 0 1 1 1 1
  spline S188 degree 3 poles (-2.7171, -13.1039) (-1.8869, -13.1039) (-1.6102, -13.1731) (-1.5237, -13.3806) knots 0 0 0 0 1 1 1 1
  spline S189 degree 3 poles (-1.5237, -13.3806) (-1.4027, -13.6919) (-2.008, -15.8539) (-2.5961, -17.1683) knots 0 0 0 0 1 1 1 1
  line L21 (-2.5961, -17.1683) -> (-2.9939, -18.085)
  line L22 (-2.9939, -18.085) -> (-4.1872, -18.1887)
  spline S190 degree 3 poles (-4.1872, -18.1887) (-9.0472, -18.6211) (-11.1573, -19.1227) (-11.2957, -19.901) knots 0 0 0 0 1 1 1 1
extrude "Extrude3" add sketch "Sketch3" along normal blind 2 bodies 1
extrude "Extrude4" add 1 faces at (-17.322, 0, -16.4132) along direction (0, -1, 0) blind 2 draft 30 on bodies 2 bodies 2
sketch "Sketch4" plane through (0, -2, 0) normal (0, -1, 0) x (1, 0, 0)
  spline S0 degree 3 poles (-7.8366, 3.3613) (-7.4734, 3.7246) (-7.1966, 3.8456) (-6.6778, 3.8456) knots 0 0 0 0 1 1 1 1
  line L0 (-6.6778, 3.8456) -> (-5.9687, 3.8456)
  line L1 (-5.9687, 3.8456) -> (-6.3319, 3.1711)
  spline S1 degree 3 poles (-6.3319, 3.1711) (-6.7988, 2.2544) (-6.7297, 1.5107) (-6.1416, 1.5107) knots 0 0 0 0 1 1 1 1
  spline S2 degree 3 poles (-6.1416, 1.5107) (-5.7957, 1.5107) (-5.7092, 1.6145) (-5.6055, 2.1161) knots 0 0 0 0 1 1 1 1
  spline S3 degree 3 poles (-5.6055, 2.1161) (-5.5363, 2.4447) (-5.2595, 2.8944) (-5.0001, 3.1192) knots 0 0 0 0 1 1 1 1
  spline S4 degree 3 poles (-5.0001, 3.1192) (-4.6196, 3.4651) (-4.3775, 3.517) (-3.5646, 3.4651) knots 0 0 0 0 1 1 1 1
  spline S5 degree 3 poles (-3.5646, 3.4651) (-2.6825, 3.4132) (-2.5961, 3.4478) (-2.5442, 3.7764) knots 0 0 0 0 1 1 1 1
  spline S6 degree 3 poles (-2.5442, 3.7764) (-2.475, 4.278) (-3.3052, 4.6066) (-4.3083, 4.5028) knots 0 0 0 0 1 1 1 1
  spline S7 degree 3 poles (-4.3083, 4.5028) (-5.7611, 4.3299) (-5.813, 4.9525) (-4.4121, 5.6962) knots 0 0 0 0 1 1 1 1
  spline S8 degree 3 poles (-4.4121, 5.6962) (-3.5646, 6.1459) (-2.4404, 6.2151) (-1.5929, 5.8519) knots 0 0 0 0 1 1 1 1
  spline S9 degree 3 poles (-1.5929, 5.8519) (-0.9876, 5.6098) (0.0847, 4.5028) (0.0847, 4.1223) knots 0 0 0 0 1 1 1 1
  spline S10 degree 3 poles (0.0847, 4.1223) (0.0847, 3.7764) (0.5171, 3.4824) (0.8457, 3.6035) knots 0 0 0 0 1 1 1 1
  spline S11 degree 3 poles (0.8457, 3.6035) (1.1916, 3.7418) (1.1916, 4.2261) (0.8457, 4.9179) knots 0 0 0 0 1 1 1 1
  spline S12 degree 3 poles (0.8457, 4.9179) (0.5863, 5.4195) (0.5863, 5.4714) (0.863, 5.6789) knots 0 0 0 0 1 1 1 1
  spline S13 degree 3 poles (0.863, 5.6789) (1.2608, 5.973) (2.7136, 6.1459) (3.4055, 6.0075) knots 0 0 0 0 1 1 1 1
  spline S14 degree 3 poles (3.4055, 6.0075) (3.7168, 5.9384) (4.2702, 5.7308) (4.6334, 5.5406) knots 0 0 0 0 1 1 1 1
  spline S15 degree 3 poles (4.6334, 5.5406) (5.2907, 5.212) (5.2907, 5.1947) (4.9966, 4.866) knots 0 0 0 0 1 1 1 1
  spline S16 degree 3 poles (4.9966, 4.866) (4.841, 4.6931) (4.5124, 4.5374) (4.2875, 4.5374) knots 0 0 0 0 1 1 1 1
  spline S17 degree 3 poles (4.2875, 4.5374) (3.7687, 4.5374) (2.8347, 4.1396) (2.5407, 3.811) knots 0 0 0 0 1 1 1 1
  spline S18 degree 3 poles (2.5407, 3.811) (2.2813, 3.4824) (2.4369, 2.9808) (2.8347, 2.9808) knots 0 0 0 0 1 1 1 1
  spline S19 degree 3 poles (2.8347, 2.9808) (2.9904, 2.9808) (3.2671, 3.1019) (3.44, 3.2403) knots 0 0 0 0 1 1 1 1
  spline S20 degree 3 poles (3.44, 3.2403) (4.2875, 3.8802) (5.9479, 3.2576) (6.2073, 2.2026) knots 0 0 0 0 1 1 1 1
  spline S21 degree 3 poles (6.2073, 2.2026) (6.2765, 1.9258) (6.4322, 1.7702) (6.6743, 1.7702) knots 0 0 0 0 1 1 1 1
  spline S22 degree 3 poles (6.6743, 1.7702) (7.4526, 1.7702) (7.2796, 2.929) (6.3803, 3.7937) knots 0 0 0 0 1 1 1 1
  line L2 (6.3803, 3.7937) -> (5.7749, 4.3472)
  line L3 (5.7749, 4.3472) -> (6.3284, 4.6412)
  spline S23 degree 3 poles (6.3284, 4.6412) (7.1931, 5.0736) (8.5941, 4.9006) (9.2686, 4.2607) knots 0 0 0 0 1 1 1 1
  spline S24 degree 3 poles (9.2686, 4.2607) (9.7702, 3.7937) (9.7702, 3.7591) (9.4243, 3.6381) knots 0 0 0 0 1 1 1 1
  spline S25 degree 3 poles (9.4243, 3.6381) (9.1648, 3.5516) (9.0783, 3.3786) (9.1129, 3.1192) knots 0 0 0 0 1 1 1 1
  spline S26 degree 3 poles (9.1129, 3.1192) (9.1648, 2.756) (9.2513, 2.7214) (9.9604, 2.7733) knots 0 0 0 0 1 1 1 1
  spline S27 degree 3 poles (9.9604, 2.7733) (11.3959, 2.8598) (12.2953, 1.7183) (11.7764, 0.473) knots 0 0 0 0 1 1 1 1
  spline S28 degree 3 poles (11.7764, 0.473) (11.6381, 0.1444) (11.3959, -0.1842) (11.2403, -0.2361) knots 0 0 0 0 1 1 1 1
  spline S29 degree 3 poles (11.2403, -0.2361) (11.1019, -0.288) (10.9808, -0.5301) (10.9808, -0.755) knots 0 0 0 0 1 1 1 1
  spline S30 degree 3 poles (10.9808, -0.755) (10.9808, -1.3603) (11.6554, -1.3084) (12.278, -0.6512) knots 0 0 0 0 1 1 1 1
  spline S31 degree 3 poles (12.278, -0.6512) (12.8487, -0.0459) (13.0563, -0.1842) (13.0563, -1.2219) knots 0 0 0 0 1 1 1 1
  spline S32 degree 3 poles (13.0563, -1.2219) (13.0563, -1.9829) (12.8487, -2.4326) (12.2261, -3.1071) knots 0 0 0 0 1 1 1 1
  spline S33 degree 3 poles (12.2261, -3.1071) (11.3959, -4.0065) (9.8566, -3.8854) (9.0092, -2.8823) knots 0 0 0 0 1 1 1 1
  spline S34 degree 3 poles (9.0092, -2.8823) (8.2655, -2.0002) (7.5218, -2.4326) (8.1098, -3.4185) knots 0 0 0 0 1 1 1 1
  spline S35 degree 3 poles (8.1098, -3.4185) (8.2655, -3.6952) (8.3865, -3.9892) (8.3865, -4.093) knots 0 0 0 0 1 1 1 1
  spline S36 degree 3 poles (8.3865, -4.093) (8.3865, -4.4216) (7.2796, -5.5458) (6.7089, -5.7706) knots 0 0 0 0 1 1 1 1
  spline S37 degree 3 poles (6.7089, -5.7706) (6.0516, -6.0474) (4.8583, -6.082) (4.4086, -5.8398) knots 0 0 0 0 1 1 1 1
  spline S38 degree 3 poles (4.4086, -5.8398) (4.0973, -5.6669) (4.0973, -5.6323) (4.5124, -5.0269) knots 0 0 0 0 1 1 1 1
  spline S39 degree 3 poles (4.5124, -5.0269) (5.0485, -4.2313) (5.0312, -3.332) (4.4951, -3.332) knots 0 0 0 0 1 1 1 1
  spline S40 degree 3 poles (4.4951, -3.332) (4.2529, -3.332) (4.0973, -3.5049) (3.9589, -3.92) knots 0 0 0 0 1 1 1 1
  spline S41 degree 3 poles (3.9589, -3.92) (3.5784, -5.1307) (2.2985, -5.5285) (1.2781, -4.7675) knots 0 0 0 0 1 1 1 1
  spline S42 degree 3 poles (1.2781, -4.7675) (0.8111, -4.4216) (0.742, -4.4043) (0.4998, -4.6637) knots 0 0 0 0 1 1 1 1
  spline S43 degree 3 poles (0.4998, -4.6637) (0.1193, -5.0442) (0.4133, -5.5285) (1.2262, -5.9263) knots 0 0 0 0 1 1 1 1
  spline S44 degree 3 poles (1.2262, -5.9263) (1.6932, -6.1511) (1.797, -6.2722) (1.624, -6.3587) knots 0 0 0 0 1 1 1 1
  spline S45 degree 3 poles (1.624, -6.3587) (1.1916, -6.6008) (0.1885, -6.6873) (-0.3304, -6.5316) knots 0 0 0 0 1 1 1 1
  spline S46 degree 3 poles (-0.3304, -6.5316) (-0.9876, -6.3241) (-1.6275, -5.7187) (-1.9215, -5.0269) knots 0 0 0 0 1 1 1 1
  spline S47 degree 3 poles (-1.9215, -5.0269) (-2.2674, -4.2313) (-2.2329, -4.1449) (-1.5929, -3.8681) knots 0 0 0 0 1 1 1 1
  spline S48 degree 3 poles (-1.5929, -3.8681) (-0.8146, -3.5568) (-0.192, -2.7612) (-0.4514, -2.4499) knots 0 0 0 0 1 1 1 1
  spline S49 degree 3 poles (-0.4514, -2.4499) (-0.7281, -2.104) (-0.9184, -2.1386) (-1.5064, -2.6402) knots 0 0 0 0 1 1 1 1
  spline S50 degree 3 poles (-1.5064, -2.6402) (-2.2328, -3.2455) (-3.0803, -3.2282) (-3.7376, -2.571) knots 0 0 0 0 1 1 1 1
  spline S51 degree 3 poles (-3.7376, -2.571) (-4.0143, -2.2943) (-4.2391, -1.9483) (-4.2391, -1.81) knots 0 0 0 0 1 1 1 1
  spline S52 degree 3 poles (-4.2391, -1.81) (-4.2391, -1.4295) (-4.7753, -1.2911) (-5.0693, -1.5851) knots 0 0 0 0 1 1 1 1
  spline S53 degree 3 poles (-5.0693, -1.5851) (-5.4671, -1.9829) (-4.7753, -3.2455) (-3.8932, -3.7471) knots 0 0 0 0 1 1 1 1
  spline S54 degree 3 poles (-3.8932, -3.7471) (-2.6479, -4.4389) (-3.2187, -5.4939) (-4.8445, -5.4939) knots 0 0 0 0 1 1 1 1
  spline S55 degree 3 poles (-4.8445, -5.4939) (-5.8476, -5.4939) (-7.1966, -4.6291) (-6.574, -4.387) knots 0 0 0 0 1 1 1 1
  spline S56 degree 3 poles (-6.574, -4.387) (-6.401, -4.3351) (-6.3146, -4.1276) (-6.3492, -3.9027) knots 0 0 0 0 1 1 1 1
  spline S57 degree 3 poles (-6.3492, -3.9027) (-6.401, -3.5568) (-6.4875, -3.5049) (-7.0929, -3.5568) knots 0 0 0 0 1 1 1 1
  spline S58 degree 3 poles (-7.0929, -3.5568) (-8.7186, -3.6606) (-9.7045, -3.1071) (-10.2233, -1.7581) knots 0 0 0 0 1 1 1 1
  spline S59 degree 3 poles (-10.2233, -1.7581) (-10.4655, -1.1009) (-10.4828, -0.876) (-10.3098, -0.3053) knots 0 0 0 0 1 1 1 1
  spline S60 degree 3 poles (-10.3098, -0.3053) (-10.0158, 0.6633) (-9.0645, 1.5626) (-8.2171, 1.701) knots 0 0 0 0 1 1 1 1
  spline S61 degree 3 poles (-8.2171, 1.701) (-7.3869, 1.8394) (-7.041, 2.168) (-7.3523, 2.5312) knots 0 0 0 0 1 1 1 1
  spline S62 degree 3 poles (-7.3523, 2.5312) (-7.4561, 2.6695) (-7.7155, 2.8079) (-7.923, 2.8425) knots 0 0 0 0 1 1 1 1
  spline S63 degree 3 poles (-7.923, 2.8425) (-8.3035, 2.8944) (-8.3035, 2.8944) (-7.8366, 3.3613) knots 0 0 0 0 1 1 1 1
  spline S64 degree 3 poles (-4.1872, -18.1887) (-9.0472, -18.6211) (-11.1573, -19.1227) (-11.2957, -19.901) knots 0 0 0 0 1 1 1 1
  spline S65 degree 3 poles (-11.2957, -19.901) (-11.5032, -20.9733) (-9.3067, -21.5613) (-3.7894, -21.9246) knots 0 0 0 0 1 1 1 1
  spline S66 degree 3 poles (-3.7894, -21.9246) (-1.0568, -22.0975) (6.6743, -21.9937) (8.9054, -21.7343) knots 0 0 0 0 1 1 1 1
  spline S67 degree 3 poles (8.9054, -21.7343) (10.9117, -21.5095) (12.7277, -21.1463) (13.3676, -20.8522) knots 0 0 0 0 1 1 1 1
  spline S68 degree 3 poles (13.3676, -20.8522) (13.9384, -20.5755) (14.0767, -19.8664) (13.627, -19.4513) knots 0 0 0 0 1 1 1 1
  spline S69 degree 3 poles (13.627, -19.4513) (13.0736, -18.967) (10.7906, -18.5346) (7.2623, -18.2406) knots 0 0 0 0 1 1 1 1
  spline S70 degree 3 poles (7.2623, -18.2406) (6.8645, -18.2233) (6.6743, -18.0504) (6.363, -17.5142) knots 0 0 0 0 1 1 1 1
  spline S71 degree 3 poles (6.363, -17.5142) (5.9825, -16.8224) (5.3425, -14.6605) (5.2388, -13.7092) knots 0 0 0 0 1 1 1 1
  spline S72 degree 3 poles (5.2388, -13.7092) (5.1869, -13.2077) (5.2215, -13.1904) (5.8787, -13.1558) knots 0 0 0 0 1 1 1 1
  spline S73 degree 3 poles (5.8787, -13.1558) (7.4872, -13.052) (9.9258, -12.7234) (10.756, -12.4813) knots 0 0 0 0 1 1 1 1
  spline S74 degree 3 poles (10.756, -12.4813) (12.1223, -12.1008) (12.3645, -11.3052) (11.3095, -10.7517) knots 0 0 0 0 1 1 1 1
  spline S75 degree 3 poles (11.3095, -10.7517) (10.756, -10.475) (8.2136, -10.0599) (6.1035, -9.8869) knots 0 0 0 0 1 1 1 1
  line L4 (6.1035, -9.8869) -> (4.7891, -9.7832)
  line L5 (4.7891, -9.7832) -> (4.7199, -8.7281)
  spline S76 degree 3 poles (4.7199, -8.7281) (4.6507, -7.431) (4.8237, -7.0505) (5.5501, -7.0505) knots 0 0 0 0 1 1 1 1
  spline S77 degree 3 poles (5.5501, -7.0505) (5.8441, -7.0505) (6.3284, -6.964) (6.6397, -6.8602) knots 0 0 0 0 1 1 1 1
  spline S78 degree 3 poles (6.6397, -6.8602) (7.0721, -6.7046) (7.2969, -6.7219) (7.7639, -6.9467) knots 0 0 0 0 1 1 1 1
  spline S79 degree 3 poles (7.7639, -6.9467) (8.5768, -7.3272) (9.7356, -7.2926) (10.4274, -6.8775) knots 0 0 0 0 1 1 1 1
  spline S80 degree 3 poles (10.4274, -6.8775) (11.05, -6.497) (11.6727, -5.5977) (11.6727, -5.0615) knots 0 0 0 0 1 1 1 1
  spline S81 degree 3 poles (11.6727, -5.0615) (11.6727, -4.8367) (11.9321, -4.5772) (12.3645, -4.3178) knots 0 0 0 0 1 1 1 1
  spline S82 degree 3 poles (12.3645, -4.3178) (14.0248, -3.3839) (14.4918, -1.3949) (13.4887, 0.3001) knots 0 0 0 0 1 1 1 1
  spline S83 degree 3 poles (13.4887, 0.3001) (12.8833, 1.3032) (12.6758, 1.9777) (12.6931, 2.7906) knots 0 0 0 0 1 1 1 1
  spline S84 degree 3 poles (12.6931, 2.7906) (12.7277, 3.6035) (12.1396, 4.745) (11.4997, 5.1082) knots 0 0 0 0 1 1 1 1
  spline S85 degree 3 poles (11.4997, 5.1082) (11.1538, 5.3157) (10.6868, 5.4195) (10.1507, 5.3849) knots 0 0 0 0 1 1 1 1
  spline S86 degree 3 poles (10.1507, 5.3849) (9.701, 5.3676) (9.1129, 5.4541) (8.8189, 5.5579) knots 0 0 0 0 1 1 1 1
  spline S87 degree 3 poles (8.8189, 5.5579) (8.5422, 5.6789) (7.8158, 5.7481) (7.245, 5.7135) knots 0 0 0 0 1 1 1 1
  spline S88 degree 3 poles (7.245, 5.7135) (6.6397, 5.6962) (6.0862, 5.7481) (5.9479, 5.8519) knots 0 0 0 0 1 1 1 1
  spline S89 degree 3 poles (5.9479, 5.8519) (5.4982, 6.2151) (4.2529, 6.7858) (3.907, 6.7858) knots 0 0 0 0 1 1 1 1
  spline S90 degree 3 poles (3.907, 6.7858) (3.7168, 6.7858) (3.2844, 7.0453) (2.9731, 7.3739) knots 0 0 0 0 1 1 1 1
  spline S91 degree 3 poles (2.9731, 7.3739) (1.624, 8.7229) (-0.0363, 8.9824) (-1.5237, 8.1176) knots 0 0 0 0 1 1 1 1
  spline S92 degree 3 poles (-1.5237, 8.1176) (-1.9907, 7.8409) (-2.4058, 7.5122) (-2.4577, 7.3739) knots 0 0 0 0 1 1 1 1
  spline S93 degree 3 poles (-2.4577, 7.3739) (-2.5096, 7.2355) (-2.7863, 7.1317) (-3.0976, 7.1317) knots 0 0 0 0 1 1 1 1
  spline S94 degree 3 poles (-3.0976, 7.1317) (-3.3916, 7.1145) (-3.9451, 6.9934) (-4.3256, 6.8377) knots 0 0 0 0 1 1 1 1
  spline S95 degree 3 poles (-4.3256, 6.8377) (-4.7061, 6.6994) (-5.3806, 6.5956) (-5.8303, 6.5956) knots 0 0 0 0 1 1 1 1
  spline S96 degree 3 poles (-5.8303, 6.5956) (-6.2973, 6.6129) (-6.9199, 6.5091) (-7.2831, 6.3362) knots 0 0 0 0 1 1 1 1
  spline S97 degree 3 poles (-7.2831, 6.3362) (-7.9749, 6.0075) (-8.7359, 5.0044) (-8.7359, 4.4164) knots 0 0 0 0 1 1 1 1
  spline S98 degree 3 poles (-8.7359, 4.4164) (-8.7359, 4.2088) (-8.8916, 3.7764) (-9.0818, 3.4651) knots 0 0 0 0 1 1 1 1
  spline S99 degree 3 poles (-9.0818, 3.4651) (-9.2721, 3.1538) (-9.4277, 2.7733) (-9.4277, 2.6349) knots 0 0 0 0 1 1 1 1
  spline S100 degree 3 poles (-9.4277, 2.6349) (-9.445, 2.4966) (-9.7391, 2.168) (-10.1023, 1.9258) knots 0 0 0 0 1 1 1 1
  spline S101 degree 3 poles (-10.1023, 1.9258) (-10.9497, 1.3205) (-11.3994, 0.3865) (-11.3994, -0.8241) knots 0 0 0 0 1 1 1 1
  spline S102 degree 3 poles (-11.3994, -0.8241) (-11.3821, -1.7927) (-10.9324, -2.9515) (-10.3963, -3.4012) knots 0 0 0 0 1 1 1 1
  spline S103 degree 3 poles (-10.3963, -3.4012) (-10.2406, -3.5395) (-10.1196, -3.8335) (-10.1196, -4.093) knots 0 0 0 0 1 1 1 1
  spline S104 degree 3 poles (-10.1196, -4.093) (-10.1023, -4.9059) (-9.4969, -5.9609) (-8.7186, -6.4797) knots 0 0 0 0 1 1 1 1
  spline S105 degree 3 poles (-8.7186, -6.4797) (-8.1306, -6.8775) (-7.802, -6.964) (-7.0237, -6.9467) knots 0 0 0 0 1 1 1 1
  spline S106 degree 3 poles (-7.0237, -6.9467) (-6.4875, -6.9467) (-5.8995, -6.8948) (-5.7092, -6.8257) knots 0 0 0 0 1 1 1 1
  spline S107 degree 3 poles (-5.7092, -6.8257) (-5.4325, -6.7219) (-5.2768, -6.8257) (-4.9828, -7.2926) knots 0 0 0 0 1 1 1 1
  spline S108 degree 3 poles (-4.9828, -7.2926) (-4.2564, -8.4168) (-2.7171, -8.8146) (-1.5064, -8.192) knots 0 0 0 0 1 1 1 1
  line L6 (-1.5064, -8.192) -> (-0.953, -7.898)
  line L7 (-0.953, -7.898) -> (-0.953, -9.7832)
  line L8 (-0.953, -9.7832) -> (-2.4577, -9.8869)
  spline S109 degree 3 poles (-2.4577, -9.8869) (-4.9309, -10.0599) (-7.6463, -10.475) (-8.1825, -10.7517) knots 0 0 0 0 1 1 1 1
  spline S110 degree 3 poles (-8.1825, -10.7517) (-9.0991, -11.236) (-9.0818, -11.8586) (-8.1133, -12.3256) knots 0 0 0 0 1 1 1 1
  spline S111 degree 3 poles (-8.1133, -12.3256) (-7.4388, -12.6369) (-4.3083, -13.1039) (-2.7171, -13.1039) knots 0 0 0 0 1 1 1 1
  spline S112 degree 3 poles (-2.7171, -13.1039) (-1.8869, -13.1039) (-1.6102, -13.1731) (-1.5237, -13.3806) knots 0 0 0 0 1 1 1 1
  spline S113 degree 3 poles (-1.5237, -13.3806) (-1.4027, -13.6919) (-2.008, -15.8539) (-2.5961, -17.1683) knots 0 0 0 0 1 1 1 1
  line L9 (-2.5961, -17.1683) -> (-2.9939, -18.085)
  line L10 (-2.9939, -18.085) -> (-4.1872, -18.1887)
  spline S114 degree 3 poles (-5.4152, -11.2187) (-4.7234, -11.1322) (-3.4608, -11.0111) (-2.6306, -10.942) knots 0 0 0 0 1 1 1 1
  line L11 (-2.6306, -10.942) -> (-1.1086, -10.8382)
  line L12 (-1.1086, -10.8382) -> (-1.1605, -11.4954)
  spline S115 degree 3 poles (-1.1605, -11.4954) (-1.2297, -12.2564) (-1.2816, -12.2737) (-3.7203, -12.0662) knots 0 0 0 0 1 1 1 1
  spline S116 degree 3 poles (-3.7203, -12.0662) (-5.9341, -11.8759) (-7.0064, -11.703) (-7.0064, -11.53) knots 0 0 0 0 1 1 1 1
  spline S117 degree 3 poles (-7.0064, -11.53) (-7.0064, -11.4435) (-6.9372, -11.3743) (-6.8507, -11.3743) knots 0 0 0 0 1 1 1 1
  spline S118 degree 3 poles (-6.8507, -11.3743) (-6.7642, -11.3743) (-6.107, -11.3052) (-5.4152, -11.2187) knots 0 0 0 0 1 1 1 1
  spline S119 degree 3 poles (10.5485, 4.3299) (10.6868, 4.4683) (11.4997, 3.8456) (11.4997, 3.5862) knots 0 0 0 0 1 1 1 1
  spline S120 degree 3 poles (11.4997, 3.5862) (11.4997, 3.223) (11.3613, 3.2576) (10.8771, 3.7937) knots 0 0 0 0 1 1 1 1
  spline S121 degree 3 poles (10.8771, 3.7937) (10.6522, 4.0359) (10.4966, 4.278) (10.5485, 4.3299) knots 0 0 0 0 1 1 1 1
  spline S122 degree 3 poles (-3.5473, -7.258) (-4.3429, -6.8775) (-4.3083, -6.5835) (-3.4435, -6.203) knots 0 0 0 0 1 1 1 1
  line L13 (-3.4435, -6.203) -> (-2.7344, -5.8744)
  line L14 (-2.7344, -5.8744) -> (-2.2674, -6.4797)
  spline S123 degree 3 poles (-2.2674, -6.4797) (-1.9907, -6.8084) (-1.8178, -7.1024) (-1.8524, -7.1197) knots 0 0 0 0 1 1 1 1
  spline S124 degree 3 poles (-1.8524, -7.1197) (-1.9907, -7.258) (-2.6825, -7.5694) (-2.8036, -7.5694) knots 0 0 0 0 1 1 1 1
  spline S125 degree 3 poles (-2.8036, -7.5694) (-2.8728, -7.5694) (-3.2187, -7.431) (-3.5473, -7.258) knots 0 0 0 0 1 1 1 1
  spline S126 degree 3 poles (9.3551, -4.6637) (9.4589, -4.5081) (10.6349, -4.8713) (10.6349, -5.0615) knots 0 0 0 0 1 1 1 1
  spline S127 degree 3 poles (10.6349, -5.0615) (10.6349, -5.6842) (9.4588, -6.3933) (8.6979, -6.2203) knots 0 0 0 0 1 1 1 1
  spline S128 degree 3 poles (8.6979, -6.2203) (8.3001, -6.1338) (8.3001, -6.0992) (8.8535, -5.3555) knots 0 0 0 0 1 1 1 1
  spline S129 degree 3 poles (8.8535, -5.3555) (9.1129, -5.0096) (9.3378, -4.6983) (9.3551, -4.6637) knots 0 0 0 0 1 1 1 1
  spline S130 degree 3 poles (-7.0237, 5.2293) (-6.5048, 5.6789) (-6.2454, 5.6789) (-6.4875, 5.2293) knots 0 0 0 0 1 1 1 1
  spline S131 degree 3 poles (-6.4875, 5.2293) (-6.5913, 5.039) (-6.8507, 4.8833) (-7.0583, 4.8833) knots 0 0 0 0 1 1 1 1
  line L15 (-7.0583, 4.8833) -> (-7.4388, 4.9006)
  line L16 (-7.4388, 4.9006) -> (-7.0237, 5.2293)
  spline S132 degree 3 poles (3.5438, -17.0645) (3.4746, -16.6494) (3.3536, -15.629) (3.2844, -14.7988) knots 0 0 0 0 1 1 1 1
  line L17 (3.2844, -14.7988) -> (3.1633, -13.2768)
  line L18 (3.1633, -13.2768) -> (3.6995, -13.2768)
  spline S133 degree 3 poles (3.6995, -13.2768) (4.1492, -13.2768) (4.2356, -13.346) (4.2356, -13.6746) knots 0 0 0 0 1 1 1 1
  spline S134 degree 3 poles (4.2356, -13.6746) (4.2356, -14.3492) (4.8929, -16.684) (5.3771, -17.7736) knots 0 0 0 0 1 1 1 1
  spline S135 degree 3 poles (5.3771, -17.7736) (5.6193, -18.3271) (6.0517, -18.9843) (6.3284, -19.2611) knots 0 0 0 0 1 1 1 1
  spline S136 degree 3 poles (6.3284, -19.2611) (6.7435, -19.6588) (6.8645, -19.6934) (7.0894, -19.5032) knots 0 0 0 0 1 1 1 1
  spline S137 degree 3 poles (7.0894, -19.5032) (7.2796, -19.3475) (7.7293, -19.3129) (8.7324, -19.3821) knots 0 0 0 0 1 1 1 1
  spline S138 degree 3 poles (8.7324, -19.3821) (10.5139, -19.5205) (12.3645, -19.8491) (12.3645, -20.0221) knots 0 0 0 0 1 1 1 1
  spline S139 degree 3 poles (12.3645, -20.0221) (12.3645, -20.195) (10.6868, -20.5063) (8.5595, -20.7139) knots 0 0 0 0 1 1 1 1
  spline S140 degree 3 poles (8.5595, -20.7139) (6.8127, -20.9041) (-1.0395, -21.0598) (-2.769, -20.956) knots 0 0 0 0 1 1 1 1
  spline S141 degree 3 poles (-2.769, -20.956) (-6.6432, -20.7139) (-9.9293, -20.2642) (-9.6526, -20.0221) knots 0 0 0 0 1 1 1 1
  spline S142 degree 3 poles (-9.6526, -20.0221) (-9.4623, -19.8491) (-7.5771, -19.5378) (-5.8822, -19.4167) knots 0 0 0 0 1 1 1 1
  spline S143 degree 3 poles (-5.8822, -19.4167) (-5.1212, -19.3475) (-4.3256, -19.2784) (-4.1181, -19.2265) knots 0 0 0 0 1 1 1 1
  spline S144 degree 3 poles (-4.1181, -19.2265) (-3.8586, -19.1746) (-3.703, -19.2611) (-3.6338, -19.5205) knots 0 0 0 0 1 1 1 1
  spline S145 degree 3 poles (-3.6338, -19.5205) (-3.5473, -19.7626) (-3.3916, -19.8491) (-3.1495, -19.8145) knots 0 0 0 0 1 1 1 1
  spline S146 degree 3 poles (-3.1495, -19.8145) (-2.6133, -19.7453) (-1.2124, -16.8743) (-0.7281, -14.8507) knots 0 0 0 0 1 1 1 1
  spline S147 degree 3 poles (-0.7281, -14.8507) (-0.3822, -13.4325) (-0.3131, -13.2768) (0.0501, -13.2768) knots 0 0 0 0 1 1 1 1
  spline S148 degree 3 poles (0.0501, -13.2768) (0.4306, -13.2768) (0.4479, -13.3287) (0.3615, -14.1935) knots 0 0 0 0 1 1 1 1
  spline S149 degree 3 poles (0.3615, -14.1935) (0.0329, -17.2894) (-0.1055, -19.3648) (-0.019, -19.5897) knots 0 0 0 0 1 1 1 1
  spline S150 degree 3 poles (-0.019, -19.5897) (0.102, -19.9356) (0.5517, -19.9183) (0.742, -19.5551) knots 0 0 0 0 1 1 1 1
  spline S151 degree 3 poles (0.742, -19.5551) (0.8284, -19.3821) (1.0014, -18.3098) (1.1052, -17.1683) knots 0 0 0 0 1 1 1 1
  spline S152 degree 3 poles (1.1052, -17.1683) (1.4684, -13.1904) (1.4684, -13.2768) (1.8316, -13.2768) knots 0 0 0 0 1 1 1 1
  spline S153 degree 3 poles (1.8316, -13.2768) (2.0045, -13.2768) (2.1602, -13.3287) (2.1602, -13.4152) knots 0 0 0 0 1 1 1 1
  spline S154 degree 3 poles (2.1602, -13.4152) (2.1602, -14.1416) (2.558, -17.5661) (2.679, -17.8774) knots 0 0 0 0 1 1 1 1
  spline S155 degree 3 poles (2.679, -17.8774) (2.852, -18.3271) (3.44, -18.4482) (3.5957, -18.0677) knots 0 0 0 0 1 1 1 1
  spline S156 degree 3 poles (3.5957, -18.0677) (3.6476, -17.9293) (3.613, -17.4969) (3.5438, -17.0645) knots 0 0 0 0 1 1 1 1
  spline S157 degree 3 poles (-0.3477, 6.2843) (-0.4341, 6.2843) (-0.7454, 6.4399) (-1.0222, 6.6129) knots 0 0 0 0 1 1 1 1
  line L19 (-1.0222, 6.6129) -> (-1.5064, 6.9242)
  line L20 (-1.5064, 6.9242) -> (-1.0741, 7.2009)
  spline S158 degree 3 poles (-1.0741, 7.2009) (-0.4168, 7.6506) (0.4479, 7.7198) (1.2089, 7.4085) knots 0 0 0 0 1 1 1 1
  spline S159 degree 3 poles (1.2089, 7.4085) (1.5721, 7.2528) (1.8143, 7.0799) (1.7624, 7.0107) knots 0 0 0 0 1 1 1 1
  spline S160 degree 3 poles (1.7624, 7.0107) (1.624, 6.8723) (-0.1228, 6.2843) (-0.3477, 6.2843) knots 0 0 0 0 1 1 1 1
  spline S161 degree 3 poles (0.4306, -11.5646) (0.4306, -12.1008) (0.3615, -12.2391) (0.1193, -12.2391) knots 0 0 0 0 1 1 1 1
  spline S162 degree 3 poles (0.1193, -12.2391) (-0.1574, -12.2391) (-0.1747, -12.1181) (-0.0363, -10.6479) knots 0 0 0 0 1 1 1 1
  spline S163 degree 3 poles (-0.0363, -10.6479) (0.0329, -9.7659) (0.0674, -8.7454) (0.0329, -8.3995) knots 0 0 0 0 1 1 1 1
  spline S164 degree 3 poles (0.0329, -8.3995) (-0.0536, -7.7769) (-0.0363, -7.7596) (0.6036, -7.6558) knots 0 0 0 0 1 1 1 1
  spline S165 degree 3 poles (0.6036, -7.6558) (1.4857, -7.5002) (1.9872, -7.8288) (1.9872, -8.5379) knots 0 0 0 0 1 1 1 1
  spline S166 degree 3 poles (1.9872, -8.5379) (1.9872, -8.8319) (2.0391, -9.7832) (2.091, -10.6479) knots 0 0 0 0 1 1 1 1
  spline S167 degree 3 poles (2.091, -10.6479) (2.2121, -12.1872) (2.1948, -12.2391) (1.8316, -12.2391) knots 0 0 0 0 1 1 1 1
  spline S168 degree 3 poles (1.8316, -12.2391) (1.5203, -12.2391) (1.4684, -12.1353) (1.4684, -11.5646) knots 0 0 0 0 1 1 1 1
  spline S169 degree 3 poles (1.4684, -11.5646) (1.4684, -10.769) (1.0879, -10.3539) (0.6901, -10.6825) knots 0 0 0 0 1 1 1 1
  spline S170 degree 3 poles (0.6901, -10.6825) (0.5344, -10.8036) (0.4306, -11.1841) (0.4306, -11.5646) knots 0 0 0 0 1 1 1 1
  spline S171 degree 3 poles (3.4746, -6.5662) (3.786, -6.7219) (3.8378, -6.8084) (3.6995, -6.9986) knots 0 0 0 0 1 1 1 1
  spline S172 degree 3 poles (3.6995, -6.9986) (3.4919, -7.2234) (2.5061, -7.3272) (2.5061, -7.1024) knots 0 0 0 0 1 1 1 1
  spline S173 degree 3 poles (2.5061, -7.1024) (2.5061, -7.0505) (2.6272, -6.8602) (2.7828, -6.6873) knots 0 0 0 0 1 1 1 1
  spline S174 degree 3 poles (2.7828, -6.6873) (3.0077, -6.4452) (3.1287, -6.4106) (3.4746, -6.5662) knots 0 0 0 0 1 1 1 1
  spline S175 degree 3 poles (3.8378, -11.0803) (3.9243, -12.1699) (3.9243, -12.2391) (3.5957, -12.2391) knots 0 0 0 0 1 1 1 1
  spline S176 degree 3 poles (3.5957, -12.2391) (3.3363, -12.2391) (3.2152, -12.0835) (3.1287, -11.703) knots 0 0 0 0 1 1 1 1
  spline S177 degree 3 poles (3.1287, -11.703) (3.0768, -11.4089) (3.025, -10.5096) (3.025, -9.714) knots 0 0 0 0 1 1 1 1
  spline S178 degree 3 poles (3.025, -9.714) (3.025, -8.3822) (3.0595, -8.2612) (3.3709, -8.2612) knots 0 0 0 0 1 1 1 1
  spline S179 degree 3 poles (3.3709, -8.2612) (3.6649, -8.2612) (3.7168, -8.3822) (3.7168, -9.0914) knots 0 0 0 0 1 1 1 1
  spline S180 degree 3 poles (3.7168, -9.0914) (3.7168, -9.541) (3.7687, -10.4231) (3.8378, -11.0803) knots 0 0 0 0 1 1 1 1
  spline S181 degree 3 poles (7.3488, -11.1149) (9.2167, -11.236) (10.1161, -11.3916) (10.1161, -11.5473) knots 0 0 0 0 1 1 1 1
  spline S182 degree 3 poles (10.1161, -11.5473) (10.1161, -11.7548) (5.1869, -12.2737) (4.9966, -12.0835) knots 0 0 0 0 1 1 1 1
  spline S183 degree 3 poles (4.9966, -12.0835) (4.962, -12.0489) (4.9275, -11.7548) (4.9275, -11.4435) knots 0 0 0 0 1 1 1 1
  spline S184 degree 3 poles (4.9275, -11.4435) (4.9275, -10.9074) (4.962, -10.8728) (5.4117, -10.942) knots 0 0 0 0 1 1 1 1
  spline S185 degree 3 poles (5.4117, -10.942) (5.6712, -10.9766) (6.5359, -11.063) (7.3488, -11.1149) knots 0 0 0 0 1 1 1 1